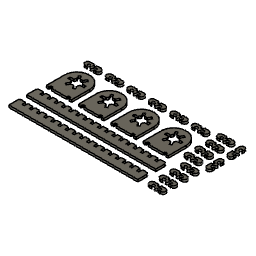
Wk6CADFrame (Autodesk Fusion 360 design; units mm, degrees)
Autodesk Fusion 360 part; units mm, degrees
note: some values were not read from the file. Set by a fixed rule: which sketch regions a step uses.
sketch "Sketch1" plane through (0, 0, 0) normal (0, 0, 1) x (1, 0, 0)
  line L0 (0, 0) -> (914.4, 0)
  line L1 (914.4, 0) -> (914.4, 76.2)
  line L2 (0, 76.2) -> (0, 0)
  line L3 (464.82, 76.2) -> (464.82, 50.8)
  line L4 (464.82, 50.8) -> (449.58, 50.8)
  line L5 (449.58, 50.8) -> (449.58, 76.2)
  line L6 (449.58, 50.8) -> (449.58, 76.2)
  line L7 (464.82, 76.2) -> (464.82, 50.8)
  line L8 (464.82, 50.8) -> (449.58, 50.8)
  line L9 (398.78, 50.8) -> (398.78, 76.2)
  line L10 (414.02, 76.2) -> (414.02, 50.8)
  line L11 (414.02, 50.8) -> (398.78, 50.8)
  line L12 (347.98, 50.8) -> (347.98, 76.2)
  line L13 (363.22, 76.2) -> (363.22, 50.8)
  line L14 (363.22, 50.8) -> (347.98, 50.8)
  line L15 (297.18, 50.8) -> (297.18, 76.2)
  line L16 (312.42, 76.2) -> (312.42, 50.8)
  line L17 (312.42, 50.8) -> (297.18, 50.8)
  line L18 (246.38, 50.8) -> (246.38, 76.2)
  line L19 (261.62, 76.2) -> (261.62, 50.8)
  line L20 (261.62, 50.8) -> (246.38, 50.8)
  line L21 (195.58, 50.8) -> (195.58, 76.2)
  line L22 (210.82, 76.2) -> (210.82, 50.8)
  line L23 (210.82, 50.8) -> (195.58, 50.8)
  line L24 (144.78, 50.8) -> (144.78, 76.2)
  line L25 (160.02, 76.2) -> (160.02, 50.8)
  line L26 (160.02, 50.8) -> (144.78, 50.8)
  line L27 (93.98, 50.8) -> (93.98, 76.2)
  line L28 (109.22, 76.2) -> (109.22, 50.8)
  line L29 (109.22, 50.8) -> (93.98, 50.8)
  line L30 (43.18, 50.8) -> (43.18, 76.2)
  line L31 (58.42, 76.2) -> (58.42, 50.8)
  line L32 (58.42, 50.8) -> (43.18, 50.8)
  line L33 (500.38, 50.8) -> (500.38, 76.2)
  line L34 (515.62, 76.2) -> (515.62, 50.8)
  line L35 (515.62, 50.8) -> (500.38, 50.8)
  line L36 (551.18, 50.8) -> (551.18, 76.2)
  line L37 (566.42, 76.2) -> (566.42, 50.8)
  line L38 (566.42, 50.8) -> (551.18, 50.8)
  line L39 (601.98, 50.8) -> (601.98, 76.2)
  line L40 (617.22, 76.2) -> (617.22, 50.8)
  line L41 (617.22, 50.8) -> (601.98, 50.8)
  line L42 (652.78, 50.8) -> (652.78, 76.2)
  line L43 (668.02, 76.2) -> (668.02, 50.8)
  line L44 (668.02, 50.8) -> (652.78, 50.8)
  line L45 (703.58, 50.8) -> (703.58, 76.2)
  line L46 (718.82, 76.2) -> (718.82, 50.8)
  line L47 (718.82, 50.8) -> (703.58, 50.8)
  line L48 (754.38, 50.8) -> (754.38, 76.2)
  line L49 (769.62, 76.2) -> (769.62, 50.8)
  line L50 (769.62, 50.8) -> (754.38, 50.8)
  line L51 (805.18, 50.8) -> (805.18, 76.2)
  line L52 (820.42, 76.2) -> (820.42, 50.8)
  line L53 (820.42, 50.8) -> (805.18, 50.8)
  line L54 (855.98, 50.8) -> (855.98, 76.2)
  line L55 (871.22, 76.2) -> (871.22, 50.8)
  line L56 (871.22, 50.8) -> (855.98, 50.8)
  line L57 (43.18, 76.2) -> (0, 76.2)
  line L58 (93.98, 76.2) -> (58.42, 76.2)
  line L59 (144.78, 76.2) -> (109.22, 76.2)
  line L60 (195.58, 76.2) -> (160.02, 76.2)
  line L61 (246.38, 76.2) -> (210.82, 76.2)
  line L62 (297.18, 76.2) -> (261.62, 76.2)
  line L63 (347.98, 76.2) -> (312.42, 76.2)
  line L64 (449.58, 76.2) -> (414.02, 76.2)
  line L65 (398.78, 76.2) -> (363.22, 76.2)
  line L66 (500.38, 76.2) -> (464.82, 76.2)
  line L67 (551.18, 76.2) -> (515.62, 76.2)
  line L68 (601.98, 76.2) -> (566.42, 76.2)
  line L69 (914.4, 76.2) -> (871.22, 76.2)
  line L70 (855.98, 76.2) -> (820.42, 76.2)
  line L71 (805.18, 76.2) -> (769.62, 76.2)
  line L72 (754.38, 76.2) -> (718.82, 76.2)
  line L73 (703.58, 76.2) -> (668.02, 76.2)
  line L74 (652.78, 76.2) -> (617.22, 76.2)
  dimension "d1" = 914.4
  dimension "d2" = 76.2
  dimension "d3" = 15.24
  dimension "d5" = 15.24
  dimension "d7" = 25.4
  dimension "d8" = 25.4
  dimension "d9" = 25.4
  dimension "d10" = 25.4
  dimension "d11" = 25.4
  dimension "d12" = 25.4
  dimension "d13" = 25.4
  dimension "d14" = 25.4
  dimension "d15" = 25.4
  dimension "d16" = 25.4
  dimension "d17" = 25.4
  dimension "d18" = 25.4
  dimension "d19" = 25.4
  dimension "d20" = 25.4
  dimension "d21" = 25.4
  dimension "d22" = 25.4
  constraint horizontal L0
  constraint vertical L2
  constraint coincident L0.start L2.end
  constraint perpendicular L4 L5
  constraint perpendicular L3 L4
  constraint perpendicular L6 L8
  constraint perpendicular L7 L8
  constraint perpendicular L10 L11
  constraint perpendicular L13 L14
  constraint perpendicular L16 L17
  constraint perpendicular L19 L20
  constraint perpendicular L22 L23
  constraint perpendicular L25 L26
  constraint perpendicular L28 L29
  constraint perpendicular L31 L32
  constraint perpendicular L34 L35
  constraint perpendicular L37 L38
  constraint perpendicular L40 L41
  constraint perpendicular L43 L44
  constraint perpendicular L46 L47
  constraint perpendicular L49 L50
  constraint perpendicular L52 L53
  constraint perpendicular L55 L56
  measures "d1" distance of L0.start L0.end
  measures "d2" distance of L0.start L2.start
  measures "d3" distance of L5.end L3.start
  measures "d5" distance of L3.start L5.end
  measures "d7" distance of L9.start L9.end
  measures "d8" distance of L12.start L12.end
  measures "d9" distance of L15.start L15.end
  measures "d10" distance of L18.start L18.end
  measures "d11" distance of L21.start L21.end
  measures "d12" distance of L24.start L24.end
  measures "d13" distance of L27.start L27.end
  measures "d14" distance of L30.start L30.end
  measures "d15" distance of L33.start L33.end
  measures "d16" distance of L36.start L36.end
  measures "d17" distance of L39.start L39.end
  measures "d18" distance of L42.start L42.end
  measures "d19" distance of L45.start L45.end
  measures "d20" distance of L48.start L48.end
  measures "d21" distance of L51.start L51.end
  measures "d22" distance of L54.start L54.end
extrude "Extrude1" add sketch "Sketch1" along normal blind 15.24 makes body 1
fillet "Fillet1" radius 12.7 2 edges at (914.4, 76.2, 7.62) (0, 76.2, 7.62) on bodies 1
fillet "Fillet2" radius 2.54 32 edges at (871.22, 76.2, 7.62) (855.98, 76.2, 7.62) (805.18, 76.2, 7.62) (820.42, 76.2, 7.62) (754.38, 76.2, 7.62) (703.58, 76.2, 7.62) (718.82, 76.2, 7.62) (668.02, 76.2, 7.62) (652.78, 76.2, 7.62) (617.22, 76.2, 7.62) (566.42, 76.2, 7.62) (500.38, 76.2, 7.62) (449.58, 76.2, 7.62) (414.02, 76.2, 7.62) (363.22, 76.2, 7.62) (297.18, 76.2, 7.62) (261.62, 76.2, 7.62) (210.82, 76.2, 7.62) (144.78, 76.2, 7.62) (160.02, 76.2, 7.62) (195.58, 76.2, 7.62) (246.38, 76.2, 7.62) (312.42, 76.2, 7.62) (347.98, 76.2, 7.62) (398.78, 76.2, 7.62) (464.82, 76.2, 7.62) (515.62, 76.2, 7.62) (551.18, 76.2, 7.62) (109.22, 76.2, 7.62) (93.98, 76.2, 7.62) (58.42, 76.2, 7.62) (43.18, 76.2, 7.62) on bodies 1
sketch "Sketch2" plane through (0, 0, 0) normal (0, 0, 1) x (1, 0, 0)
  line L0 (88.9, 508) -> (88.9, 381)
  line L1 (-88.9, 381) -> (-88.9, 508)
  line L2 (-54.61, 381) -> (-54.61, 393.7)
  line L3 (-54.61, 393.7) -> (-69.85, 393.7)
  line L4 (-69.85, 393.7) -> (-69.85, 381)
  line L5 (54.61, 381) -> (54.61, 393.7)
  line L6 (54.61, 393.7) -> (69.85, 393.7)
  line L7 (69.85, 393.7) -> (69.85, 381)
  line L8 (-56.9595, 515.62) -> (-30.6258, 515.62)
  line L9 (-30.6258, 500.38) -> (-56.9595, 500.38)
  line L10 (-56.9595, 500.38) -> (-56.9595, 515.62)
  line L11 (-35.0789, 462.4816) -> (-21.912, 485.2873)
  line L12 (-21.8806, 454.8616) -> (-35.0789, 462.4816)
  line L13 (-8.7138, 477.6673) -> (-21.8806, 454.8616)
  line L14 (21.8806, 454.8616) -> (8.7138, 477.6673)
  line L15 (35.0789, 462.4816) -> (21.8806, 454.8616)
  line L16 (21.912, 485.2873) -> (35.0789, 462.4816)
  line L17 (56.9595, 500.38) -> (30.6258, 500.38)
  line L18 (56.9595, 515.62) -> (56.9595, 500.38)
  line L19 (30.6258, 515.62) -> (56.9595, 515.62)
  line L20 (35.0789, 553.5184) -> (21.912, 530.7127)
  line L21 (21.8806, 561.1384) -> (35.0789, 553.5184)
  line L22 (8.7138, 538.3327) -> (21.8806, 561.1384)
  line L23 (-21.8806, 561.1384) -> (-8.7138, 538.3327)
  line L24 (-35.0789, 553.5184) -> (-21.8806, 561.1384)
  line L25 (-21.912, 530.7127) -> (-35.0789, 553.5184)
  arc A0 (-21.912, 530.7127) -> (-30.6258, 515.62) centre (0, 508) ccw
  arc A1 (8.7138, 538.3327) -> (-8.7138, 538.3327) centre (0, 508) ccw
  arc A2 (30.6258, 515.62) -> (21.912, 530.7127) centre (0, 508) ccw
  arc A3 (21.912, 485.2873) -> (30.6258, 500.38) centre (0, 508) ccw
  arc A4 (-30.6258, 500.38) -> (-21.912, 485.2873) centre (0, 508) ccw
  arc A5 (-8.7138, 477.6673) -> (8.7138, 477.6673) centre (0, 508) ccw
  arc A6 (88.9, 507.9846) -> (-88.9, 508) centre (0, 508) ccw
  line L26 (88.9, 381) -> (69.85, 381)
  line L27 (54.61, 381) -> (-54.61, 381)
  line L28 (-69.85, 381) -> (-88.9, 381)
  dimension "d29" = 63.119
  dimension "d30" = 177.8
  dimension "d31" = 15.24
  dimension "d32" = 12.7
  dimension "d33" = 15.24
  dimension "d34" = 12.7
  dimension "d35" = 19.05
  dimension "d36" = 19.05
  dimension "d39" = 15.24
  dimension "d42" = 360
  constraint concentric A4 A6
  constraint vertical L0
  constraint horizontal L26
  constraint vertical L1
  constraint vertical L2
  constraint horizontal L3
  constraint vertical L4
  constraint coincident L4.end L26
  constraint vertical L5
  constraint horizontal L6
  constraint vertical L7
  constraint horizontal L8
  constraint horizontal L9
  constraint vertical L10
  constraint concentric A0 A4
  constraint concentric A1 A4
  constraint concentric A2 A4
  constraint concentric A3 A4
  constraint concentric A4 A5
  constraint coincident L0 A6.start
  constraint collinear L26 L27
  constraint collinear L27 L28
  measures "d29" diameter of A4
  measures "d30" diameter of A6
  measures "d31" distance of L4.end L2.start
  measures "d32" distance of L4.end L3.end
  measures "d33" distance of L7.end L5.start
  measures "d34" distance of L7.end L6.end
  measures "d35" distance of L1 L4
  measures "d36" distance of L0 L7
  measures "d39" distance of L8.start L9.end
extrude "Extrude2" add sketch "Sketch2" along normal blind 15.24 separate body makes body 2
fillet "Fillet3" radius 2.54 16 edges at (-30.6258, 515.62, 7.62) (-21.912, 530.7127, 7.62) (-8.7138, 538.3327, 7.62) (8.7138, 538.3327, 7.62) (21.912, 530.7127, 7.62) (30.6258, 515.62, 7.62) (30.6258, 500.38, 7.62) (21.912, 485.2873, 7.62) (8.7138, 477.6673, 7.62) (-8.7138, 477.6673, 7.62) (-21.912, 485.2873, 7.62) (-30.6258, 500.38, 7.62) (-69.85, 381, 7.62) (-54.61, 381, 7.62) (54.61, 381, 7.62) (69.85, 381, 7.62) on bodies 2
sketch "Sketch3" plane through (0, 0, 0) normal (0, 0, 1) x (1, 0, 0)
  arc A0 (330.2, 361.95) -> (330.2, 400.05) centre (330.2, 381) ccw
  arc A1 (254, 400.05) -> (254, 361.95) centre (254, 381) ccw
  line L0 (299.72, 400.05) -> (299.72, 387.35)
  line L1 (299.72, 387.35) -> (284.48, 387.35)
  line L2 (284.48, 387.35) -> (284.48, 400.05)
  line L3 (254, 400.05) -> (284.48, 400.05)
  line L4 (299.72, 400.05) -> (330.2, 400.05)
  spline S0 degree 5 poles (266.7739, 361.95) (267.3445, 361.9215) (268.4048, 361.8871) (269.7523, 361.904) (271.0628, 362.0632) (271.9013, 362.4858) (271.9755, 363.1174) (271.3587, 363.9284) (270.1774, 364.8678) (268.5942, 365.8749) (266.7885, 366.8915) (264.9377, 367.8753) (263.1992, 368.8105) (261.6889, 369.7248) (260.477, 370.6823) (259.6005, 371.7556) (259.071, 373.003) (258.8837, 374.4465) (259.0266, 376.0425) (259.4827, 377.6966) (260.2287, 379.2913) (261.235, 380.7102) (262.465, 381.8608) (263.8747, 382.7044) (265.4152, 383.2495) (267.0365, 383.532) (268.6916, 383.5989) (270.3395, 383.4928) (271.9503, 383.2311) (273.5033, 382.8085) (274.984, 382.2081) (276.3796, 381.4107) (277.6772, 380.4041) (278.8581, 379.1941) (279.9016, 377.8054) (280.791, 376.2755) (281.5199, 374.6503) (282.0982, 372.9795) (282.5588, 371.3122) (282.9609, 369.6928) (283.3784, 368.1607) (283.8907, 366.7496) (284.5732, 365.4873) (285.4871, 364.3943) (286.6716, 363.4836) (288.1497, 362.7627) (289.576, 362.3406) (290.7842, 362.1114) (291.6511, 361.9973) (292.1, 361.95) knots 0 0 0 0 0 0 0.022222 0.044444 0.066667 0.088889 0.111111 0.133333 0.155556 0.177778 0.2 0.222222 0.244444 0.266667 0.288889 0.311111 0.333333 0.355556 0.377778 0.4 0.422222 0.444444 0.466667 0.488889 0.511111 0.533333 0.555556 0.577778 0.6 0.622222 0.644444 0.666667 0.688889 0.711111 0.733333 0.755556 0.777778 0.8 0.822222 0.844444 0.866667 0.888889 0.911111 0.933333 0.955556 0.977778 1 1 1 1 1 1
  spline S1 degree 5 poles (317.4261, 361.95) (316.8555, 361.9215) (315.7952, 361.8871) (314.4478, 361.904) (313.1372, 362.0632) (312.2987, 362.4858) (312.2245, 363.1174) (312.8413, 363.9284) (314.0226, 364.8678) (315.6058, 365.8749) (317.4115, 366.8915) (319.2623, 367.8753) (321.0008, 368.8105) (322.5111, 369.7248) (323.723, 370.6823) (324.5995, 371.7556) (325.129, 373.003) (325.3163, 374.4465) (325.1734, 376.0425) (324.7173, 377.6966) (323.9713, 379.2913) (322.965, 380.7102) (321.735, 381.8608) (320.3253, 382.7044) (318.7848, 383.2495) (317.1635, 383.5319) (315.5084, 383.5989) (313.8605, 383.4928) (312.2497, 383.2311) (310.6967, 382.8085) (309.2161, 382.2081) (307.8204, 381.4107) (306.5229, 380.4041) (305.3419, 379.1941) (304.2984, 377.8054) (303.409, 376.2755) (302.6801, 374.6502) (302.1018, 372.9795) (301.6412, 371.3122) (301.2391, 369.6928) (300.8216, 368.1606) (300.3093, 366.7496) (299.6268, 365.4873) (298.7129, 364.3943) (297.5285, 363.4836) (296.0503, 362.7627) (294.624, 362.3406) (293.4158, 362.1114) (292.5489, 361.9973) (292.1, 361.95) knots 0 0 0 0 0 0 0.022222 0.044444 0.066667 0.088889 0.111111 0.133333 0.155556 0.177778 0.2 0.222222 0.244444 0.266667 0.288889 0.311111 0.333333 0.355556 0.377778 0.4 0.422222 0.444444 0.466667 0.488889 0.511111 0.533333 0.555556 0.577778 0.6 0.622222 0.644444 0.666667 0.688889 0.711111 0.733333 0.755556 0.777778 0.8 0.822222 0.844444 0.866667 0.888889 0.911111 0.933333 0.955556 0.977778 1 1 1 1 1 1
  line L5 (253.8839, 362.5951) -> (279.6639, 361.3049)
  line L6 (284.3491, 362.7672) -> (299.851, 361.1328)
  line L7 (330.3161, 362.5951) -> (304.5361, 361.3049)
  line L8 (299.851, 362.7672) -> (284.3491, 361.1328)
  line L9 (254, 361.95) -> (269.7157, 361.95)
  line L10 (292.1, 361.95) -> (292.1001, 361.95)
  line L11 (314.4846, 361.95) -> (330.2, 361.95)
  point P0 (271.78, 363.22)
  point P1 (264.16, 368.3)
  point P2 (259.08, 373.38)
  point P3 (261.62, 381)
  point P4 (269.24, 383.54)
  point P5 (276.86, 381)
  point P6 (281.94, 373.38)
  point P7 (284.48, 365.76)
  point P8 (312.42, 363.22)
  point P9 (320.04, 368.3)
  point P10 (325.12, 373.38)
  point P11 (322.58, 381)
  point P12 (314.96, 383.54)
  point P13 (307.34, 381)
  point P14 (302.26, 373.38)
  point P15 (299.72, 365.76)
  dimension "d48" = 38.1
  dimension "d49" = 15.24
  dimension "d50" = 12.7
  dimension "d51" = 30.48
  dimension "d52" = 30.48
  constraint tangent A0 L3
  constraint tangent A0 L9
  constraint tangent A1 L3
  constraint tangent A1 L9
  constraint vertical L0
  constraint horizontal L1
  constraint vertical L2
  constraint collinear L3 L4
  constraint midpoint S0.start L5
  constraint midpoint S0.end L6
  constraint coincident S0 L9.end
  constraint coincident S0 S1.end
  constraint collinear L9 L10
  constraint coincident S0.end L9
  constraint coincident S1 L10.end
  constraint coincident S1 L11.start
  constraint collinear L10 L11
  measures "d48" diameter of A0
  measures "d49" distance of L2.end L0.start
  measures "d50" distance of L2.end L1.end
  measures "d51" distance of A0.end L0
  measures "d52" distance of A1.start L2
extrude "Extrude3" add sketch "Sketch3" along normal blind 15.24 separate body contours A0 A1 L0 L1 L2 L3 L4 S0 S1 L9 L11 makes body 3
fillet "Fillet4" radius 2.54 2 edges at (284.48, 400.05, 7.62) (299.72, 400.05, 7.62) on bodies 3
move_body "Move1" bodies 1 to x (1, 0, 0) y (0, 1, 0) z (0, 0, 1) at (25.4, 25.4, 0)
copy_body "CopyPasteBodies1" bodies 1 makes body 4
move_body "Move2" bodies 4 to x (1, 0, 0) y (0, 1, 0) z (0, 0, 1) at (0, 127, 0)
move_body "Move3" bodies 3 to x (1, 0, 0) y (0, 1, 0) z (0, 0, 1) at (0, 330.2, 0)
move_body "Move4" bodies 2 to x (1, 0, 0) y (0, 1, 0) z (0, 0, 1) at (127, -101.6, 0)
copy_body "CopyPasteBodies2" bodies 2 makes body 5
move_body "Move5" bodies 5 to x (1, 0, 0) y (0, 1, 0) z (0, 0, 1) at (228.6, 0, 0)
copy_body "CopyPasteBodies3" bodies 2 makes body 6
move_body "Move6" bodies 6 to x (1, 0, 0) y (0, 1, 0) z (0, 0, 1) at (457.2, 0, 0)
copy_body "CopyPasteBodies4" bodies 2 makes body 7
move_body "Move7" bodies 7 to x (1, 0, 0) y (0, 1, 0) z (0, 0, 1) at (685.8, 0, 0)
copy_body "CopyPasteBodies10" bodies 3 makes body 8
move_body "Move17" bodies 8 to x (1, 0, 0) y (0, 1, 0) z (0, 0, 1) at (152.4, -0.0001, 0)
move_body "Move18" bodies 8 to x (1, 0, 0) y (0, 1, 0) z (0, 0, 1) at (609.5996, -660.4004, 0)
copy_body "CopyPasteBodies11" bodies 8 makes body 9
move_body "Move19" bodies 9 to x (1, 0, 0) y (0, 1, 0) z (0, 0, 1) at (0, 76.2, 0)
copy_body "CopyPasteBodies12" bodies 8 9 makes body 10 makes body 11
move_body "Move20" bodies 10 11 to x (1, 0, 0) y (0, 1, 0) z (0, 0, 1) at (0, 152.4, 0)
copy_body "CopyPasteBodies13" bodies 11 10 makes body 12 makes body 13
move_body "Move21" bodies 12 13 to x (1, 0, 0) y (0, 1, 0) z (0, 0, 1) at (-50.7999, 152.4, 0)
move_body "Move22" bodies 3 to x (1, 0, 0) y (0, 1, 0) z (0, 0, 1) at (-203.2, -152.4, 0)
copy_body "CopyPasteBodies14" bodies 3 makes body 14
move_body "Move23" bodies 14 to x (1, 0, 0) y (0, 1, 0) z (0, 0, 1) at (152.4, 0, 0)
copy_body "CopyPasteBodies15" bodies 3 14 makes body 15 makes body 16
move_body "Move24" bodies 15 16 to x (1, 0, 0) y (0, 1, 0) z (0, 0, 1) at (304.8, -0.0001, 0)
copy_body "CopyPasteBodies17" bodies 15 16 makes body 17 makes body 18
move_body "Move26" bodies 17 18 to x (1, 0, 0) y (0, 1, 0) z (0, 0, 1) at (304.8, 0, 0)
copy_body "CopyPasteBodies18" bodies 13 12 makes body 19 makes body 20
move_body "Move27" bodies 19 20 to x (1, 0, 0) y (0, 1, 0) z (0, 0, 1) at (0, 152.4, 0)
copy_body "CopyPasteBodies19" bodies 20 makes body 21
move_body "Move28" bodies 21 to x (0, 1, 0) y (-1, 0, 0) z (0, 0, 1) at (1701.7993, -457.2001, 0)
copy_body "CopyPasteBodies20" bodies 21 makes body 22
move_body "Move29" bodies 22 to x (1, 0, 0) y (0, 1, 0) z (0, 0, 1) at (-0.0001, -152.4, 0)
